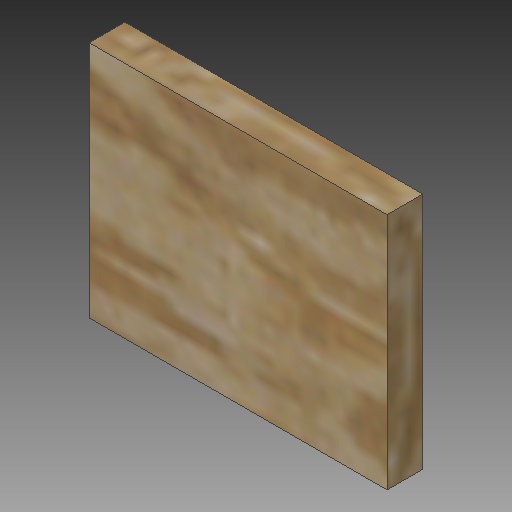
# Autodesk Inventor part: 3_4 Intake Board
Saved by Autodesk Inventor 2018 (Build 220112000, 112)
## iProperties
Created: 2018-01-17
Part Number: 3_4 Intake Board
Material: Generic
Document SubType Name: Modeling
Designer: Apple
Density: 1 g/cm^3
Appearance: Plywood - Weathered
Author: Apple
Autodesk Inventor part; units mm, degrees
ref_plane "YZ Plane" through (0, 0, 0) normal (1, 0, 0) x (0, 1, 0)
ref_plane "XZ Plane" through (0, 0, 0) normal (0, 1, 0) x (-1, 0, 0)
ref_plane "XY Plane" through (0, 0, 0) normal (0, 0, 1) x (1, 0, 0)
sketch "Sketch1" plane through (0, 0, 0) normal (0, 0, 1) x (1, 0, 0)
  line L0 (793.75, -38.7488) -> (635, -38.7488)
  line L1 (635, -38.7488) -> (635, 88.2512)
  line L2 (635, 88.2512) -> (793.75, 88.2512)
  line L3 (793.75, 88.2512) -> (793.75, -38.7488)
  line L4 (793.75, 73.787) -> (793.75, 3.937) projected
  line L5 (684.0312, 142.2262) -> (788.5674, 142.2262) construction
  line L6 (787.4, 81.407) -> (622.3, 81.407) construction
  point P0 (0, 0)
  point P1 (793.75, 24.7512)
  point P2 (793.75, 38.862)
  dimension "d0" = 158.75
  dimension "d2" = 60.8192
  dimension "d3" = 180.975
  dimension "d4" = 127
  constraints: 10 end point, 2 horizontal, 2 midpoint, 2 parallel, 1 perpendicular, 1 vertical alignment
  measures "d0" distance of L0.start L0.end
  measures "d2" distance between parallel lines of L6 L5
  measures "d3" distance between parallel lines of L0 L5
  measures "d4" distance of L2.end L0.start
extrude "Extrusion1" add sketch "Sketch1" along normal blind 19.05
body "Solid1"
